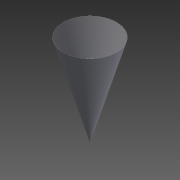
# Autodesk Inventor part: cone
Saved by Autodesk Inventor 2015 (Build 190159000, 159)
## iProperties
Created: 2015-08-16
Part Number: cone
Material: Generic
Document SubType Name: Modeling
Designer: Burton1
Density: 1 g/cm^3
Appearance: Default
Author: Burton1
Autodesk Inventor part; units mm, degrees
ref_plane "YZ Plane" through (0, 0, 0) normal (1, 0, 0) x (0, 1, 0)
ref_plane "XZ Plane" through (0, 0, 0) normal (0, 1, 0) x (-1, 0, 0)
ref_plane "XY Plane" through (0, 0, 0) normal (0, 0, 1) x (1, 0, 0)
sketch "Sketch1" plane through (0, 0, 0) normal (0, 0, 1) x (1, 0, 0)
  line L0 (1371.6, -350.5424) -> (1371.6, 5034.3551)
  line L1 (0, 4724.4) -> (1371.6, 4724.4)
  line L2 (1371.6, 0) -> (0, 4724.4)
  point P0 (0, 0)
  constraints: 6 end point, 2 point on line, 1 horizontal, 1 vertical
revolve "Revolution1" add sketch "Sketch1" angle 360 about axis through (1371.6, -350.5424, 0) along (0, 1, 0)
shell "Shell1" thickness 6.35 removed faces 1 at (938.5915, 4724.4, 51.3525)
body "Solid1"
